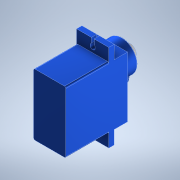
# Autodesk Inventor part: Servomotor HTX900
Saved by Autodesk Inventor 2021 (Build 250183000, 183)
## iProperties
Created: 2016-01-04
Part Number: Servomotor HTX900
Material: Поликарбонат, дымчатый
Document SubType Name: Modeling
Designer: Evgeny
Density: 1.2 g/cm^3
Appearance: Анодированный — синий
Author: Evgeny
Autodesk Inventor part; units mm, degrees
ref_plane "YZ Plane" through (0, 0, 0) normal (1, 0, 0) x (0, 1, 0)
ref_plane "XZ Plane" through (0, 0, 0) normal (0, 1, 0) x (-1, 0, 0)
sketch "Эскиз1" plane through (0, 0, 0) normal (0, 1, 0) x (-1, 0, 0)
  line L0 (5.5, 11.5) -> (-5.5, 11.5)
  line L1 (-6, 11) -> (-6, -11)
  line L2 (-5.5, -11.5) -> (5.5, -11.5)
  line L3 (6, -11) -> (6, 11)
  line L4 (6, 11.5) -> (-6, -11.5) construction
  line L5 (-6, 11.5) -> (6, -11.5) construction
  arc A0 (6, 11) -> (5.5, 11.5) centre (5.5, 11) ccw
  arc A1 (5.5, -11.5) -> (6, -11) centre (5.5, -11) ccw
  arc A2 (-6, -11) -> (-5.5, -11.5) centre (-5.5, -11) ccw
  arc A3 (-5.5, 11.5) -> (-6, 11) centre (-5.5, 11) ccw
  point P0 (0, 0)
  dimension "d0" = 12
  dimension "d1" = 23
  dimension "d2" = 0.5
  constraints: 12 end point, 8 point on circle, 8 point on line, 8 tangent, 4 centre point, 3 equal radius, 2 midpoint, 2 parallel, 1 horizontal, 1 perpendicular
  measures "d0" distance of L5.end L4.end
  measures "d1" distance of L4.end L5.start
  measures "d2" radius of A0
extrude "Выдавливание1" add sketch "Эскиз1" along normal blind 16
sketch "Эскиз2" plane through (0, 16, 0) normal (0, 1, 0) x (1, 0, 0)
  line L0 (6, -16.25) -> (6, 16.25)
  line L1 (-6, 16.25) -> (-6, -16.25)
  line L2 (-6, -16.25) -> (6, 16.25) construction
  line L3 (6, -16.25) -> (-6, 16.25) construction
  arc A0 (0.5, -14.366) -> (-0.5, -14.366) centre (0, -13.5) ccw
  arc A1 (-0.5, 14.366) -> (0.5, 14.366) centre (0, 13.5) ccw
  line L4 (-0.5, -14.366) -> (-0.5, -16.25)
  line L5 (0.5, -14.366) -> (0.5, -16.25)
  line L6 (-6, -16.25) -> (-0.5, -16.25)
  line L7 (0.5, -16.25) -> (6, -16.25)
  line L8 (-0.5, 14.366) -> (-0.5, 16.25)
  line L9 (0.5, 14.366) -> (0.5, 16.25)
  line L10 (6, 16.25) -> (0.5, 16.25)
  line L11 (-0.5, 16.25) -> (-6, 16.25)
  point P0 (0, 0)
  point P1 (0, 0)
  point P2 (0, 0)
  dimension "d5" = 12
  dimension "d6" = 32.5
  dimension "d7" = 2
  dimension "d8" = 2
  dimension "d9" = 1
  dimension "d10" = 0.5
  dimension "d13" = 27
  dimension "d14" = 13.5
  constraints: 24 end point, 10 perpendicular, 5 parallel, 4 midpoint, 4 point on circle, 2 centre point, 2 collinear, 2 horizontal, 1 vertical alignment
  measures "d5" distance of L1.start L0.end
  measures "d6" distance of L0.end L0.start
  measures "d7" diameter of A0
  measures "d8" diameter of A1
  measures "d9" distance between parallel lines of L5 L4
  measures "d10" distance from line of L4 A0.centre
  measures "d13" distance of A1.centre A0.centre
  measures "d14" distance of point (0, 0) A0.centre
extrude "Выдавливание2" add sketch "Эскиз2" along normal blind 2
sketch "Эскиз3" plane through (0, 18, 0) normal (0, 1, 0) x (1, 0, 0)
  line L0 (6, -16.25) -> (6, 16.25) projected
  line L1 (-6, -11.25) -> (6, -11.25)
  line L2 (6, -11.25) -> (6, 11.25)
  line L3 (6, 11.25) -> (-6, 11.25)
  line L4 (-6, 11.25) -> (-6, -11.25)
  line L5 (-6, -11.25) -> (6, 11.25) construction
  line L6 (6, -11.25) -> (-6, 11.25) construction
  point P0 (0, 0)
  dimension "d15" = 22.5
  dimension "d18" = 12
  constraints: 12 end point, 2 midpoint, 2 parallel, 1 horizontal, 1 perpendicular, 1 point on line
  measures "d15" distance of L2.end L1.end
  measures "d18" distance of L2.end L3.end
extrude "Выдавливание3" add sketch "Эскиз3" along normal blind 5
sketch "Эскиз4" plane through (0, 23, 0) normal (0, 1, 0) x (1, 0, 0)
  arc A0 (-2.75, -0.2002) -> (2.75, -0.2002) centre (0, -5.25) ccw
  arc A1 (2.75, 0.75) -> (-2.75, 0.75) centre (0, 0.75) ccw
  line L0 (-2.75, 0.75) -> (-2.75, -0.2002)
  line L1 (2.75, 0.75) -> (2.75, -0.2002)
  line L2 (-6, -11.25) -> (6, -11.25) projected
  point P0 (0, 0)
  dimension "d19" = 11.5
  dimension "d20" = 5.25
  dimension "d21" = 5.5
  dimension "d22" = 6
  dimension "d23" = 11.25
  constraints: 4 end point, 4 point on circle, 2 centre point, 2 tangent, 2 vertical, 2 vertical alignment
  measures "d19" diameter of A0
  measures "d20" distance of A0.centre point (0, 0)
  measures "d21" diameter of A1
  measures "d22" distance of A1.centre A0.centre
  measures "d23" distance from line of point (0, 0) L2
extrude "Выдавливание4" add sketch "Эскиз4" along normal blind 4
fillet "Сопряжение1" radius 0.25 4 edges at (0, 27, 11) (0, 27, -3.5) (2.75, 27, -0.2749) (-2.75, 27, -0.2749)
sketch "Эскиз5" plane through (0, 23, 0) normal (0, 1, 0) x (1, 0, 0)
  line L0 (-4.25, 4.75) -> (4.25, 4.75)
  line L1 (4.5, 5) -> (4.5, 9.5)
  line L2 (4.25, 9.75) -> (-4.25, 9.75)
  line L3 (-4.5, 9.5) -> (-4.5, 5)
  line L4 (6, 11.25) -> (-6, 11.25) projected
  line L5 (-6, 11.25) -> (-6, -11.25) projected
  line L6 (6, -11.25) -> (6, 11.25) projected
  arc A0 (-4.5, 5) -> (-4.25, 4.75) centre (-4.25, 5) ccw
  arc A1 (-4.25, 9.75) -> (-4.5, 9.5) centre (-4.25, 9.5) ccw
  arc A2 (4.5, 9.5) -> (4.25, 9.75) centre (4.25, 9.5) ccw
  arc A3 (4.25, 4.75) -> (4.5, 5) centre (4.25, 5) ccw
  point P0 (0, 0)
  dimension "d27" = 1.5
  dimension "d28" = 1.5
  dimension "d29" = 1.5
  dimension "d30" = 5
  dimension "d31" = 0.25
  constraints: 8 end point, 8 point on circle, 8 tangent, 4 centre point, 3 equal radius, 2 parallel, 1 horizontal, 1 perpendicular
  measures "d27" distance between parallel lines of L2 L4
  measures "d28" distance between parallel lines of L3 L5
  measures "d29" distance between parallel lines of L6 L1
  measures "d30" distance between parallel lines of L0 L2
  measures "d31" radius of A0
extrude "Выдавливание5" cut sketch "Эскиз5" against normal blind 0.25
sketch "Эскиз6" plane through (0, 27, 0) normal (0, 1, 0) x (1, 0, 0)
  arc A0 (-2.5, -0.351) -> (2.5, -0.351) centre (0, -5.25) ccw projected
  circle A1 centre (0, -5.25) radius 2.25
  circle A2 centre (0, -5.25) radius 0.5
  point P0 (0, 0)
  dimension "d34" = 4.5
  dimension "d35" = 1
  constraints: 2 centre point, 2 coincident
  measures "d34" diameter of A1
  measures "d35" diameter of A2
extrude "Выдавливание6" add sketch "Эскиз6" along normal blind 3
ref_plane "Work Plane1" through (0, 0, 11) normal (1, 0, 0) x (0, 0, -1)
equation "\"d8\" = d7"
equation "\"d14\" = 0.5 * d13"
equation "\"d28\" = d27"
equation "\"d29\" = d27"
equation "\"d45\" = 0.5 * d44"
equation "\"d44\" = 0.8"
